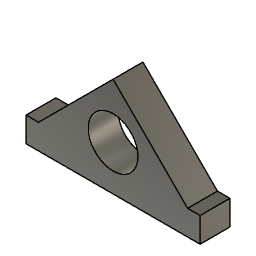
Sorter v3 (Autodesk Fusion 360 design; units mm, degrees)
Autodesk Fusion 360 part; units mm, degrees
note: some values were not read from the file. Set by a fixed rule: which sketch regions a step uses.
sketch "Sketch1" plane through (0, 0, 0) normal (0, 1, 0) x (1, 0, 0)
  line L0 (-22.2401, 0) -> (22.2401, 0)
  line L1 (22.2401, 0) -> (22.2401, 6.35)
  line L2 (22.2401, 6.35) -> (-22.2401, 6.35)
  line L3 (-22.2401, 6.35) -> (-22.2401, 0)
  line L4 (0, 0) -> (0, -19.05)
  line L5 (0, -19.05) -> (-19.05, 0)
  line L6 (0, -19.05) -> (-21.997, -19.05) construction
  line L7 (0, -19.05) -> (19.05, 0)
  dimension "d1" = 19.05
  dimension "d2" = 45
  dimension "d6" = 25.4
  constraint horizontal L0
  constraint vertical L1
  constraint horizontal L2
  constraint vertical L3
  constraint midpoint L4.start L0
  constraint coincident L4.start origin
  constraint perpendicular L0 L4
  constraint horizontal L6
  constraint coincident L0 L5.end
  constraint symmetric L5.start L4 L6.start
  constraint symmetric L4 L5.end L7.end
  measures "d1" distance of L4.start L4.end
  measures "d2" angle of L5 L6
  measures "d6" distance of L2 L4.end
extrude "Extrude1" add sketch "Sketch1" along normal blind 7.62
sketch "Sketch2" plane through (0, 0, 0) normal (0, -1, 0) x (1, 0, 0)
  line L0 (19.05, 0) -> (0, 19.05)
  line L1 (0, 19.05) -> (-19.05, 0)
  line L2 (-19.05, 0) -> (-22.2401, 0)
  line L3 (-22.2401, 0) -> (-22.2401, -6.35)
  line L4 (-22.2401, -6.35) -> (22.2401, -6.35)
  line L5 (22.2401, -6.35) -> (22.2401, 0)
  line L6 (22.2401, 0) -> (19.05, 0)
  line L7 (0, -6.35) -> (0, 20.8829)
  circle A0 centre (0, 5.08) radius 6.35
  dimension "d12" = 12.7
  constraint midpoint L4 L7.start
  constraint perpendicular L4 L7
  constraint coincident L7 A0.centre
  measures "d12" diameter of A0
extrude "Extrude2" cut sketch "Sketch2" against normal blind 54.61 contours L7 A0 | L7 A0
equation "d1 = triangleHeight"
equation "d2 = triangleDeg"
equation "length = 1 in"
equation "height = 1 in"
equation "triangleHeight = 0.75 in"
equation "d6 = height"
equation "triangleDeg = 45 deg"
equation "width = 0.3 in"
equation "d9 = width"
equation "AxleHoleDia = 0.5 in"
equation "d12 = AxleHoleDia"
